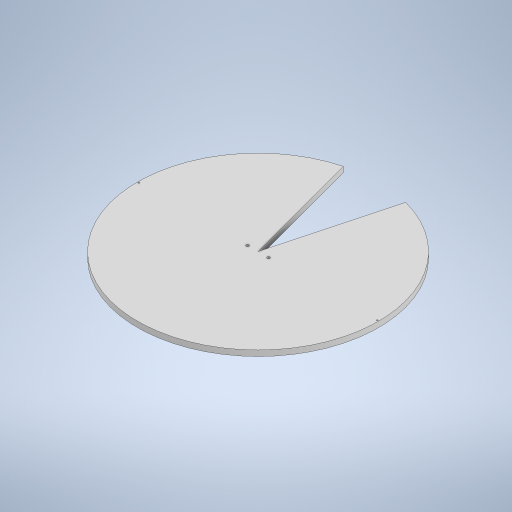
# Autodesk Inventor part: seed_disp_lid
Saved by Autodesk Inventor 2023 (Build 270158000, 158)
## iProperties
Created: 2022-06-19
Part Number: seed_disp_lid
Material: Generic
Document SubType Name: Modeling
Designer: prana_p9lsmih
Density: 1 g/cm^3
Appearance: Default
Author: prana_p9lsmih
Autodesk Inventor part; units mm, degrees
ref_plane "YZ Plane" through (0, 0, 0) normal (1, 0, 0) x (0, 1, 0)
ref_plane "XY Plane" through (0, 0, 0) normal (0, 0, 1) x (1, 0, 0)
sketch "Sketch1" plane through (0, 0, 0) normal (0, 1, 0) x (-1, 0, 0)
  arc A0 (11.1292, -41.5348) -> (-11.1292, -41.5348) centre (0, 0) ccw
  line L0 (0, 0) -> (11.1292, -41.5348)
  line L1 (0, 0) -> (43, 0) construction
  line L2 (0, 0) -> (-11.1292, -41.5348)
  dimension "d0" = 86
  dimension "d1" = 75
  constraints: 6 end point, 2 point on circle, 1 centre point, 1 coincident, 1 equal length, 1 horizontal
  measures "d0" diameter of A0
  measures "d1" angle of L0 L1
extrude "Extrusion1" add sketch "Sketch1" along normal blind 2
ref_plane "Work Plane1" through (0, 1, 0) normal (0, 1, 0) x (-1, 0, 0)
sketch "Sketch2" plane through (0, 2, 0) normal (0, 1, 0) x (1, 0, 0)
  circle A0 centre (-42.5, 0) radius 0.25
  arc A1 (-11.1292, 41.5348) -> (11.1292, 41.5348) centre (0, 0) ccw projected
  dimension "d4" = 0.5
  dimension "d5" = 42.5
  constraints: 1 centre point
  measures "d4" diameter of A0
  measures "d5" distance of A0.centre A1.centre
extrude "Extrusion2" cut sketch "Sketch2" against normal through all
mirror "Mirror1" about plane through (0, 0, 0) normal (1, 0, 0) of "Extrusion2"
sketch "Sketch4" plane through (0, 2, 0) normal (0, 1, 0) x (1, 0, 0)
  circle A0 centre (-3.75, 0) radius 0.5
  point P0 (0, 0)
  dimension "d12" = 1
  dimension "d13" = 3.75
  constraints: 1 centre point
  measures "d12" diameter of A0
  measures "d13" distance of point (0, 0) A0.centre
extrude "Extrusion4" cut sketch "Sketch4" against normal through all
mirror "Mirror3" about plane through (0, 0, 0) normal (1, 0, 0) of "Extrusion4"
body "Solid1"
